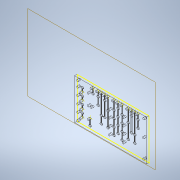
# Autodesk Inventor part: Control Layer
Saved by Autodesk Inventor 2021 (Build 250183000, 183)
## iProperties
Created: 2020-06-07
Part Number: Control Layer
Material: Generic
Document SubType Name: Modeling
Designer: natha
Density: 1 g/cm^3
Appearance: Default
Author: natha
Autodesk Inventor part; units mm, degrees
ref_plane "YZ Plane" through (0, 0, 0) normal (1, 0, 0) x (0, 1, 0)
ref_plane "XZ Plane" through (0, 0, 0) normal (0, 1, 0) x (-1, 0, 0)
sketch "Sketch1" plane through (0, 0, 0) normal (0, 0, 1) x (1, 0, 0)
  line L0 (-177, 0) -> (-177, 100) projected
  line L1 (-177, 100) -> (0, 100) projected
  line L2 (0, 100) -> (0, 0) projected
  line L3 (0, 0) -> (-177, 0) projected
extrude "Extrusion base plate" add sketch "Sketch1" along normal blind 6
ref_plane "work plane for rib creation" through (0, 0, -1) normal (0, 0, 1) x (1, 0, 0)
sketch3d "channels and points for valves and for connectors for contro"
  constraints: 44 end point, 17 coincident, 15 vertical, 5 parallel, 5 point on line, 2 perpendicular, 1 horizontal, 15 other
sketch "channels and points for valves and for connectors for control layer" plane through (0, 0, -1) normal (0, 0, 1) x (1, 0, 0)
  line L0 (0, 0) -> (-300, 0) construction
  line L1 (-300, 0) -> (-300, 200) construction
  line L2 (-300, 200) -> (0, 200) construction
  line L3 (0, 200) -> (0, 0) construction
  line L4 (-300, 23) -> (0, 23) construction
  line L5 (0, 92) -> (-300, 92) construction
  line L6 (-26, 61) -> (-26, 92)
  line L7 (-34, 25) -> (-34, 92)
  line L8 (-42, 43) -> (-42, 92)
  line L9 (-50, 25) -> (-50, 92)
  line L10 (-65, 16) -> (-65, 92)
  line L11 (-75, 25) -> (-75, 92)
  line L12 (-85, 16) -> (-85, 92)
  line L13 (-100, 25) -> (-100, 92)
  line L14 (-108, 43) -> (-108, 92)
  line L15 (-116, 25) -> (-116, 92)
  line L16 (-124, 61) -> (-124, 92)
  line L17 (-137, 79) -> (-137, 92)
  line L18 (-144, 7) -> (-144, 23)
  line L19 (-163, 25) -> (-163, 16)
  line L20 (-163, 43) -> (-163, 34)
  line L21 (-163, 61) -> (-163, 52)
  line L22 (-163, 79) -> (-163, 70)
  line L23 (0, 100) -> (-177, 100)
  point P0 (-124, 79)
  point P1 (-116, 43)
  point P2 (-108, 79)
  point P3 (-100, 61)
  point P4 (-85, 34)
  point P5 (-85, 52)
  point P6 (-85, 70)
  point P7 (-75, 79)
  point P8 (-75, 61)
  point P9 (-75, 43)
  point P10 (-65, 34)
  point P11 (-65, 52)
  point P12 (-65, 70)
  point P13 (-50, 61)
  point P14 (-42, 79)
  point P15 (-34, 43)
  point P16 (-26, 79)
rib "channels as rib" sketch "channels and points for valves and for connectors for control layer" thickness 1 direction (0, 0, 1) end up to next extend profile no curves L19 L20 L21 L22 L18 L17 L16 L15 L13 L14 L12 L11 L10 L9 L8 L7 L6
sketch "Sketch3" plane through (-162.5, 70, -1) normal (0, 0, -1) x (-1, 0, 0)
  line L0 (1, 0) -> (0, 0) projected
  line L1 (1, 9) -> (1, 0) projected
  line L2 (0, 9) -> (1, 9) projected
  line L3 (0, 0) -> (0, 9) projected
  line L4 (1, -18) -> (0, -18) projected
  line L5 (1, -9) -> (1, -18) projected
  line L6 (0, -9) -> (1, -9) projected
  line L7 (0, -18) -> (0, -9) projected
  line L8 (1, -36) -> (0, -36) projected
  line L9 (1, -27) -> (1, -36) projected
  line L10 (0, -27) -> (1, -27) projected
  line L11 (0, -36) -> (0, -27) projected
  line L12 (1, -54) -> (0, -54) projected
  line L13 (1, -45) -> (1, -54) projected
  line L14 (0, -45) -> (1, -45) projected
  line L15 (0, -54) -> (0, -45) projected
  line L16 (-19, -47) -> (-18, -47) projected
  line L17 (-19, -63) -> (-19, -47) projected
  line L18 (-18, -63) -> (-19, -63) projected
  line L19 (-18, -47) -> (-18, -63) projected
  line L20 (-26, 9) -> (-26, 22) projected
  line L21 (-25, 22) -> (-25, 9) projected
  line L22 (-26, 22) -> (-25, 22) projected
  line L23 (-26, 9) -> (-26, 22) projected
  line L24 (-25, 9) -> (-26, 9) projected
  line L25 (-25, 22) -> (-25, 9) projected
  line L26 (-39, 22) -> (-38, 22) projected
  line L27 (-39, -9) -> (-39, 22) projected
  line L28 (-38, -9) -> (-39, -9) projected
  line L29 (-38, 22) -> (-38, -9) projected
  line L30 (-47, 22) -> (-46, 22) projected
  line L31 (-47, -45) -> (-47, 22) projected
  line L32 (-46, -45) -> (-47, -45) projected
  line L33 (-46, 22) -> (-46, -45) projected
  line L34 (-55, 22) -> (-54, 22) projected
  line L35 (-55, -27) -> (-55, 22) projected
  line L36 (-54, -27) -> (-55, -27) projected
  line L37 (-54, 22) -> (-54, -27) projected
  line L38 (-63, 22) -> (-62, 22) projected
  line L39 (-63, -45) -> (-63, 22) projected
  line L40 (-62, -45) -> (-63, -45) projected
  line L41 (-62, 22) -> (-62, -45) projected
  line L42 (-78, 22) -> (-77, 22) projected
  line L43 (-78, -54) -> (-78, 22) projected
  line L44 (-77, -54) -> (-78, -54) projected
  line L45 (-77, 22) -> (-77, -54) projected
  line L46 (-88, 22) -> (-87, 22) projected
  line L47 (-88, -45) -> (-88, 22) projected
  line L48 (-87, -45) -> (-88, -45) projected
  line L49 (-87, 22) -> (-87, -45) projected
  line L50 (-98, 22) -> (-97, 22) projected
  line L51 (-98, -54) -> (-98, 22) projected
  line L52 (-97, -54) -> (-98, -54) projected
  line L53 (-97, 22) -> (-97, -54) projected
  line L54 (-113, 22) -> (-112, 22) projected
  line L55 (-113, -45) -> (-113, 22) projected
  line L56 (-112, -45) -> (-113, -45) projected
  line L57 (-112, 22) -> (-112, -45) projected
  line L58 (-121, 22) -> (-120, 22) projected
  line L59 (-121, -27) -> (-121, 22) projected
  line L60 (-120, -27) -> (-121, -27) projected
  line L61 (-120, 22) -> (-120, -27) projected
  line L62 (-129, 22) -> (-128, 22) projected
  line L63 (-129, -45) -> (-129, 22) projected
  line L64 (-128, -45) -> (-129, -45) projected
  line L65 (-128, 22) -> (-128, -45) projected
  line L66 (-137, 22) -> (-136, 22) projected
  line L67 (-137, -9) -> (-137, 22) projected
  line L68 (-136, -9) -> (-137, -9) projected
  line L69 (-136, 22) -> (-136, -9) projected
  point P0 (-162.5, -70)
  point P1 (-26, 22)
extrude "extrusion of ribs to get cutout" cut sketch "Sketch3" against normal blind 2.6
sketch "Sketch4" plane through (0, 0, 0) normal (0, 0, 1) x (1, 0, 0)
  ellipse E0 centre (-65, 16) end of major axis (-62.5, 16) minor radius 1.75 projected
  ellipse E1 centre (-65, 16) end of major axis (-62, 16) minor radius 2.25
  point P0 (0, 0)
  dimension "d50" = 3
  dimension "d51" = 2.25
  constraints: 1 centre point
extrude "valve space extrusion" cut sketch "Sketch4" along normal blind 1.6 contours E0 | E1
pattern_sketch "all valve spaces" of "valve space extrusion" from (-65, 16, 0) copies at (-26, 61, 0) at (-26, 79, 0) at (-34, 43, 0) at (-34, 25, 0) at (-42, 43, 0) at (-42, 79, 0) at (-50, 61, 0) at (-50, 25, 0) at (-65, 34, 0) at (-65, 52, 0) at (-65, 70, 0) at (-75, 79, 0) at (-75, 61, 0) at (-75, 43, 0) at (-75, 25, 0) at (-85, 16, 0) at (-85, 34, 0) at (-85, 52, 0) at (-85, 70, 0) at (-100, 61, 0) at (-100, 25, 0) at (-108, 43, 0) at (-108, 79, 0) at (-116, 43, 0) at (-116, 25, 0) at (-124, 61, 0) at (-124, 79, 0) at (-137, 79, 0) at (-144, 7, 0) at (-163, 25, 0) at (-163, 43, 0) at (-163, 61, 0) at (-163, 79, 0)
sketch "projected points for every hole for control layer only" plane through (0, 0, 0) normal (0, 0, 1) x (1, 0, 0)
  point P0 (0, 0)
  point P1 (-163, 70)
  point P2 (-163, 52)
  point P3 (-163, 34)
  point P4 (-163, 16)
  point P5 (-144, 23)
  point P6 (-137, 92)
  point P7 (-137, 92)
  point P8 (-124, 92)
  point P9 (-116, 92)
  point P10 (-108, 92)
  point P11 (-100, 92)
  point P12 (-85, 92)
  point P13 (-75, 92)
  point P14 (-65, 92)
  point P15 (-50, 92)
  point P16 (-42, 92)
  point P17 (-34, 92)
  point P18 (-34, 92)
  point P19 (-26, 92)
hole "holes for control layer" at (-26, 92, 0) at (-34, 92, 0) at (-42, 92, 0) at (-50, 92, 0) at (-65, 92, 0) at (-75, 92, 0) at (-85, 92, 0) at (-100, 92, 0) at (-108, 92, 0) at (-116, 92, 0) at (-124, 92, 0) at (-137, 92, 0) at (-163, 16, 0) at (-163, 34, 0) at (-163, 52, 0) at (-163, 70, 0) at (-144, 23, 0) direction (0, 0, 1) diameter 4.2 depth 6
sketch "projected points for every hole for flow layer only" plane through (0, 0, 0) normal (0, 0, 1) x (1, 0, 0)
  point P0 (0, 0)
  point P1 (-170, 25)
  point P2 (-170, 43)
  point P3 (-170, 61)
  point P4 (-170, 79)
  point P5 (-144, 79)
  point P6 (-144, 52)
  point P7 (-137, 52)
  point P8 (-92, 16)
  point P9 (-92, 34)
  point P10 (-92, 52)
  point P11 (-92, 70)
  point P12 (-58, 70)
  point P13 (-58, 52)
  point P14 (-58, 34)
  point P15 (-58, 16)
  point P16 (-8, 52)
hole "holes for connection to flow layer" at (-8, 52, 0) at (-58, 16, 0) at (-58, 34, 0) at (-58, 52, 0) at (-58, 70, 0) at (-92, 70, 0) at (-92, 52, 0) at (-92, 34, 0) at (-92, 16, 0) at (-137, 52, 0) at (-144, 52, 0) at (-144, 79, 0) at (-170, 61, 0) at (-170, 43, 0) at (-170, 25, 0) at (-170, 79, 0) direction (0, 0, 1) diameter 4.2 depth 6
sketch "projection for holes in corners" plane through (0, 0, 0) normal (0, 0, 1) x (1, 0, 0)
  point P0 (0, 0)
  point P1 (-170, 93)
  point P2 (-170, 7)
  point P3 (-7, 7)
  point P4 (-7, 93)
hole "holes in corners" at (-170, 7, 0) at (-170, 93, 0) at (-7, 7, 0) at (-7, 93, 0) direction (0, 0, 1) diameter 4.5 end through all
sketch "Projected points for every valve" plane through (0, 0, 0) normal (0, 0, 1) x (1, 0, 0)
  point P0 (0, 0)
  point P1 (-26, 61)
  point P2 (-26, 79)
  point P3 (-34, 43)
  point P4 (-34, 25)
  point P5 (-42, 43)
  point P6 (-42, 79)
  point P7 (-50, 61)
  point P8 (-50, 25)
  point P9 (-65, 16)
  point P10 (-65, 34)
  point P11 (-65, 52)
  point P12 (-65, 70)
  point P13 (-75, 79)
  point P14 (-75, 61)
  point P15 (-75, 43)
  point P16 (-75, 25)
  point P17 (-85, 16)
  point P18 (-85, 34)
  point P19 (-85, 52)
  point P20 (-85, 70)
  point P21 (-100, 61)
  point P22 (-100, 25)
  point P23 (-108, 43)
  point P24 (-108, 79)
  point P25 (-116, 43)
  point P26 (-116, 25)
  point P27 (-124, 61)
  point P28 (-124, 79)
  point P29 (-137, 79)
  point P30 (-144, 7)
  point P31 (-163, 25)
  point P32 (-163, 43)
  point P33 (-163, 61)
  point P34 (-163, 79)
equation "\"d10\" = d9"
equation "\"d11\" = d9"
equation "\"d12\" = d9"
equation "\"d27\" = engraving_depth"
equation "\"engraving_depth\" = 1.6"
equation "\"d9\" = 9"
body "Solid1"
